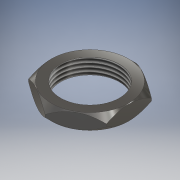
# Autodesk Inventor part: Ecrou plug alimentation
Saved by Autodesk Inventor 2017 (Build 210142000, 142)
## iProperties
Company: FABLAB Frenchmakers
Part Number: Ecrou plug alimentation
Project: 1420 VAUBAN 3D XL
Material: ----------
Catalog Web Link: http://www.frenchmakers.com/
Document SubType Name: Modeling
Designer: FABLAB Frenchmakers
Mass: 0.593859 g
Surface Area: 1.81123 cm^2
Volume: 0.0755546 cm^3
Density: 7.86 g/cm^3
Appearance: Acier - Poli
Stock Number: 1420-09-03
Autodesk Inventor part; units mm, degrees
ref_plane "YZ Plane" through (0, 0, 0) normal (1, 0, 0) x (0, 1, 0)
ref_plane "XZ Plane" through (0, 0, 0) normal (0, 1, 0) x (-1, 0, 0)
ref_plane "XY Plane" through (0, 0, 0) normal (0, 0, 1) x (1, 0, 0)
sketch "Esquisse1" plane through (0, 0, 0) normal (0, 0, 1) x (1, 0, 0)
  line L0 (4.94, 2.8521) -> (4.94, -2.8521)
  line L1 (4.94, -2.8521) -> (0, -5.7042)
  line L2 (0, -5.7042) -> (-4.94, -2.8521)
  line L3 (-4.94, -2.8521) -> (-4.94, 2.8521)
  line L4 (-4.94, 2.8521) -> (0, 5.7042)
  line L5 (0, 5.7042) -> (4.94, 2.8521)
  point P0 (0, 0)
  point P1 (0, 0)
  dimension "d0" = 9.88
  constraints: 12 end point, 1 coincident, 1 vertical, 13 other
  measures "d0" distance between parallel lines of L0 L3
extrude "Extrusion1" add sketch "Esquisse1" along normal mid plane 1.96
sketch "Esquisse2" plane through (0, 0, 0.98) normal (0, 0, 1) x (1, 0, 0)
  point P0 (0, 0)
  point P1 (0, 0)
  constraints: 1 coincident
hole "Perçage1" at (0, 0, 0.98) direction (0, 0, -1) diameter 7.459 depth 18.8 tip angle 118 thread size "M8x0.5" class "6H" standard "ISO Metric profile"
sketch "Esquisse3" plane through (0, 0, 0) normal (0, 1, 0) x (-1, 0, 0)
  line L0 (-4.94, 0.98) -> (0, 0.98) construction
  line L1 (-4.94, -0.98) -> (-4.94, 0.98) construction
  line L2 (-3.94, 1.93) -> (-5.94, -0.07)
  line L3 (-5.94, -0.07) -> (-5.94, 1.93)
  line L4 (-5.94, 1.93) -> (-3.94, 1.93)
  line L5 (0, -1.432) -> (0, 1.732) projected
  point P0 (0, 0)
  point P1 (-4.89, 0.98)
  point P2 (-4.94, 0.93)
  point P3 (-4.94, 1.93)
  dimension "d12" = 0.05
  dimension "d13" = 0.05
  dimension "d14" = 2
  constraints: 6 end point, 3 point on line, 2 midpoint, 1 horizontal, 1 vertical, 1 vertical alignment
  measures "d12" distance from line of L1 point (-4.89, 0.98)
  measures "d13" distance from line of point (-4.94, 0.93) L0
  measures "d14" distance of L3.end L2.start
revolve "Révolution1" cut sketch "Esquisse3" angle 360 about axis through (0, 0, -10) along (0, 0, 1)
mirror "Symétrie1" about plane through (0, 0, 0) normal (0, 0, 1) of "Révolution1"
equation "\"d13\" = d12"
